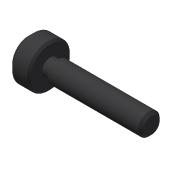
# Autodesk Inventor part: Screw Adjust
Saved by Autodesk Inventor 2022 Beta2 (Build 260130000, 130) ContinuousBuild 0
## iProperties
Created: 2006-01-31
Part Number: Screw Adjust
Document SubType Name: Modeling
Designer: landrews
Stock Number: Screw Adjust
Density: 1 g/cm^3
Material: Generic
Appearance: Generic
Author: landrews
Autodesk Inventor part; units mm, degrees
ref_plane "YZ Plane" through (0, 0, 0) normal (1, 0, 0) x (0, 1, 0)
ref_plane "XZ Plane" through (0, 0, 0) normal (0, 1, 0) x (-1, 0, 0)
ref_plane "XY Plane" through (0, 0, 0) normal (0, 0, 1) x (1, 0, 0)
sketch "Sketch1" plane through (0, 0, 0) normal (0, 1, 0) x (-1, 0, 0)
  line L0 (-59.15, 0) -> (4.55, 0) projected
  line L1 (0, -0.8) -> (0, 10.4) projected
  line L2 (0, 0) -> (0, 6)
  line L3 (0, 6) -> (-2, 8)
  line L4 (-2, 8) -> (-7.2929, 8)
  line L5 (-7.2929, 8) -> (-8, 7.2929)
  line L6 (-8, 7.2929) -> (-8, 3.05)
  line L7 (-8, 3.05) -> (-10.5, 3.05)
  line L8 (-10.5, 3.05) -> (-11.0485, 4)
  line L9 (-11.0485, 4) -> (-44.5, 4)
  line L10 (-44.5, 4) -> (-45.5, 3)
  line L11 (-45.5, 3) -> (-45.5, 0)
  line L12 (-45.5, 0) -> (0, 0)
  dimension "d0" = 2
  dimension "d1" = 8
  dimension "d2" = 45
  dimension "d3" = 8
  dimension "d5" = 2.5
  dimension "d6" = 3.05
  dimension "d8" = 1
  dimension "d10" = 4
  dimension "d11" = 45.5
  dimension "d12" = 2
  dimension "d13" = 60
  dimension "d14" = 1
  dimension "d15" = 1
  constraints: 22 end point, 4 perpendicular, 4 point on line, 1 collinear, 1 parallel
  measures "d0" horizontal distance of L2.end L3.end
  measures "d1" distance between parallel lines of L0 L4
  measures "d2" angle of L4 L5
  measures "d3" distance between parallel lines of L6 L1
  measures "d5" distance of L6.end L7.end
  measures "d6" distance between parallel lines of L12 L7
  measures "d8" horizontal distance of L9.end L10.end
  measures "d10" distance between parallel lines of L12 L9
  measures "d11" distance between parallel lines of L1 L11
  measures "d12" horizontal distance of L2.end L3.end
  measures "d13" angle of L9 L8
  measures "d14" distance of L4.end L5.end
  measures "d15" horizontal distance of L9.end L10.end
revolve "Revolution1" add sketch "Sketch1" angle 360 about axis through (45.5, 0, 0) along (-1, 0, 0)
body "Solid1"
